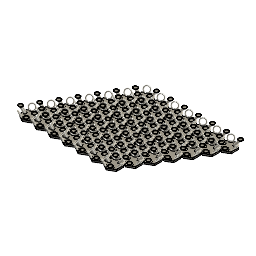
Week 5 3D Print (Autodesk Fusion 360 design; units mm, degrees)
part number: 2025-10-03-17-33-42-323
Autodesk Fusion 360 part; units mm, degrees
sketch "Sketch1" plane through (0, 0, 0) normal (0, 0, 1) x (1, 0, 0)
  line L0 (2.101, 5.3776) -> (-3.6067, 4.5083)
  line L1 (-3.6067, 4.5083) -> (-5.7077, -0.8693)
  line L2 (-5.7077, -0.8693) -> (-2.101, -5.3776)
  line L3 (-2.101, -5.3776) -> (3.6067, -4.5083)
  line L4 (3.6067, -4.5083) -> (5.7077, 0.8693)
  line L5 (5.7077, 0.8693) -> (2.101, 5.3776)
  dimension "d1" = 10
  measures "d1" distance of L1 L4
torus "TorusPrimitive1" add centre line diameter 4.2 section diameter 1 placed x (-1, 0, 0) y (0, -1, 0) z (0, 0, 1) at (1.5, 2, 1.2) makes body 1
delete_face "DeleteFace1" 1 faces at (1.8195, 4.5499, 1.371) on bodies 1
sketch "Sketch3" plane through (0, 0, 0) normal (0, 0, 1) x (1, 0, 0)
  line L0 (5, 2.8868) -> (0, 5.7735)
  line L1 (0, 5.7735) -> (-5, 2.8868)
  line L2 (-5, 2.8868) -> (-5, -2.8868)
  line L3 (-5, -2.8868) -> (0, -5.7735)
  line L4 (0, -5.7735) -> (5, -2.8868)
  line L5 (5, -2.8868) -> (5, 2.8868)
  dimension "d6" = 10
  measures "d6" distance of L2 L5
extrude "Extrude2" add sketch "Sketch3" along normal blind 1.2 separate body makes body 2
torus "TorusPrimitive2" add centre line diameter 4.2 section diameter 1 placed x (-1, 0, 0) y (0, -1, 0) z (0, 0, 1) at (1.6402, 2.114, 1.2) separate body makes body 3
move_body "MoveFace1" bodies 3 to x (0, 0, 1) y (0, 1, 0) z (-1, 0, 0) at (2.8402, 0, -0.4402) on bodies 3
move_body "MoveFace2" bodies 3 to x (0.866025, 0, -0.5) y (0, 1, 0) z (0.5, 0, 0.866025) at (2.4797, -2.1, 2.9809) on bodies 3
move_body "MoveFace3" bodies 3 to x (1, 0, 0) y (0, 1, 0) z (0, 0, 1) at (1.0532, 0, -0.0593) on bodies 3
pattern_circular "C-Pattern1" count 3 over 360 about axis through (0, 0, 1.75) along (0, 0, 1) of bodies 3 makes body 4 at (-4.8085, 4.4471, 4.6988) makes body 5 at (-4.9641, -4.0524, 4.2415)
sketch "Sketch5" plane through (0, 0, 1.2) normal (0, 0, 1) x (-1, 0, 0)
  line L0 (-5, 2.8868) -> (-5, -2.8868)
  line L1 (-5, -2.8868) -> (0, -5.7735)
  line L2 (0, -5.7735) -> (5, -2.8868)
  line L3 (5, -2.8868) -> (5, 2.8868)
  line L4 (5, 2.8868) -> (0, 5.7735)
  line L5 (0, 5.7735) -> (-5, 2.8868)
  circle A0 centre (-1.875, 3.2476) radius 1.25
  line L6 (0, 0) -> (-2.5, 4.3301) construction
  circle A1 centre (-1.875, -3.2476) radius 1.25
  circle A2 centre (3.75, 0) radius 1.25
  line L7 (-2.5, 4.3301) -> (-4.5483, 7.8778) construction
  dimension "d13" = 2.5
  dimension "d15" = 360
  constraint coincident L6.start origin
  constraint midpoint L5 L6.end
  constraint coincident A0.centre L6
  constraint tangent L5 A0
  constraint perpendicular L5 L7
  measures "d13" diameter of A0
ref_plane "WorkPlane1" through (0, 0, 4.4) normal (0, 0, 1) x (-1, 0, 0)
sketch "Sketch6" plane through (0, 0, 4.4) normal (0, 0, 1) x (1, 0, 0)
  circle A0 centre (3.4995, -6.0625) radius 1.25
  circle A1 centre (3.5005, 6.0619) radius 1.25
  circle A2 centre (-7, 0.0005) radius 1.25
  point P0 (1.875, -3.2476)
  dimension "d17" = 2.5
  dimension "d18" = 3.25
  dimension "d20" = 360
  measures "d17" diameter of A0
  measures "d18" distance of A0.centre P0
loft "Loft1" add profiles "Sketch6", "Sketch5" section 1 contours A0 section 2 contours A0 bodies 2
loft "Loft2" add profiles "Sketch5", "Sketch6" section 1 contours A1 section 2 contours A1 bodies 2
loft "Loft3" add profiles "Sketch5", "Sketch6" section 1 contours A2 section 2 contours A2 bodies 2
sketch "Sketch7" plane through (0, 0, 4.4) normal (0, 0, 1) x (1, 0, 0)
  circle A0 centre (3.5005, 6.0619) radius 1.65
  circle A1 centre (3.5005, 6.0619) radius 1.25
  circle A2 centre (-7, 0.0005) radius 1.65
  circle A3 centre (3.4995, -6.0625) radius 1.65
  dimension "d21" = 3.3
  dimension "d23" = 360
  constraint concentric A0 A1
  measures "d21" diameter of A0
extrude "Extrude3" add sketch "Sketch7" sketch "Sketch6" along normal blind 0.3 of sketch 2 contours A0 | A1 bodies 2
combine "Combine1" operation add target body 2 tool bodies 3 5 4
sketch "Sketch8" plane through (0, 0, 1.2) normal (0, 0, 1) x (-1, 0, 0)
  line L0 (0, 0) -> (-10.7359, -18.5415) construction
  line L1 (0, 0) -> (-18.5422, 0) construction
  constraint coincident L0.start L1.start
  constraint horizontal L1
pattern_linear "R-Pattern1" count 7 spacing 11 along (1, 0, 0) count 7 spacing 11 along (0.501082, 0.8654, 0) of bodies 2 makes body 6 at (11, 0, 0) makes body 7 at (23.6667, 0.9623, 0) makes body 8 at (31.3333, 0.9623, 0) makes body 9 at (42.3333, 0.9623, 0) makes body 10 at (53.3333, 0.9623, 0) makes body 11 at (64.3333, 0.9623, 0) makes body 12 at (3.8452, 8.5571, 0) makes body 13 at (16.5119, 7.5949, 0) makes body 14 at (25.8452, 8.5571, 0) makes body 15 at (36.8452, 10.4816, 0) makes body 16 at (47.8452, 10.4816, 0) makes body 17 at (58.8452, 10.4816, 0) makes body 18 at (69.8452, 10.4816, 0) makes body 19 at (9.3571, 20.001, 0) makes body 20 at (23.6905, 18.0765, 0) makes body 21 at (33.0238, 17.1143, 0) makes body 22 at (42.3571, 20.001, 0) makes body 23 at (53.3571, 20.001, 0) makes body 24 at (64.3571, 20.001, 0) makes body 25 at (75.3571, 20.001, 0) makes body 26 at (18.2024, 29.5204, 0) makes body 27 at (27.5357, 30.4827, 0) makes body 28 at (40.2024, 27.5959, 0) makes body 29 at (51.2024, 27.5959, 0) makes body 30 at (62.2024, 27.5959, 0) makes body 31 at (73.2024, 27.5959, 0) makes body 32 at (84.2024, 27.5959, 0) makes body 33 at (22.0476, 36.1531, 0) makes body 34 at (33.0476, 38.0776, 0) makes body 35 at (42.3809, 37.1153, 0) makes body 36 at (53.3809, 37.1153, 0) makes body 37 at (64.3809, 37.1153, 0) makes body 38 at (75.3809, 37.1153, 0) makes body 39 at (86.3809, 37.1153, 0) makes body 40 at (27.5595, 45.6725, 0) makes body 41 at (36.8928, 46.6347, 0) makes body 42 at (47.8928, 46.6347, 0) makes body 43 at (58.8928, 46.6347, 0) makes body 44 at (69.8928, 46.6347, 0) makes body 45 at (80.8928, 46.6347, 0) makes body 46 at (91.8928, 46.6347, 0) makes body 47 at (33.0714, 57.1164, 0) makes body 48 at (44.0714, 57.1164, 0) makes body 49 at (55.0714, 57.1164, 0) makes body 50 at (66.0714, 57.1164, 0) makes body 51 at (77.0714, 57.1164, 0) makes body 52 at (88.0714, 57.1164, 0) makes body 53 at (99.0714, 57.1164, 0)
